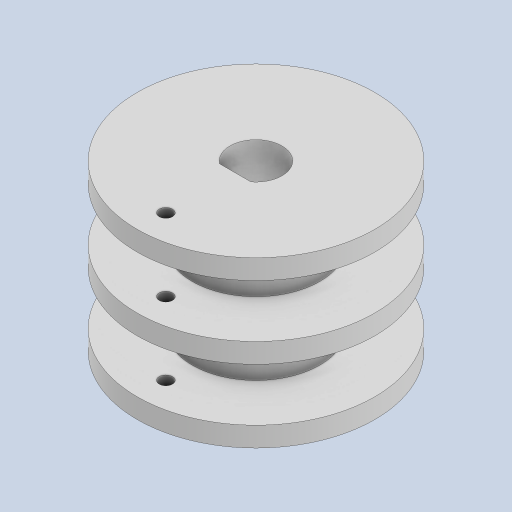
# Autodesk Inventor part: PulleyV2
Saved by Autodesk Inventor 2024 (Build 280153000, 153)
## iProperties
Created: 2024-01-01
Part Number: PulleyV2
Material: Generic
Document SubType Name: Modeling
Designer: Greg
Density: 1 g/cm^3
Appearance: Default
Author: Greg
Autodesk Inventor part; units mm, degrees
ref_plane "YZ Plane" through (0, 0, 0) normal (1, 0, 0) x (0, 1, 0)
ref_plane "XZ Plane" through (0, 0, 0) normal (0, 1, 0) x (-1, 0, 0)
ref_plane "XY Plane" through (0, 0, 0) normal (0, 0, 1) x (1, 0, 0)
sketch "Sketch1" plane through (0, 0, 0) normal (0, 1, 0) x (-1, 0, 0)
  circle A0 centre (0, 0) radius 14.2875
  dimension "d0" = 28.575
  constraints: 1 centre point, 1 coincident
  measures "d0" diameter of A0
extrude "Extrusion1" add sketch "Sketch1" along normal blind 2.3813
sketch "Sketch2" plane through (0, 2.3813, 0) normal (0, 1, 0) x (1, 0, 0)
  circle A0 centre (0, 0) radius 6.096 construction
  circle A1 centre (0, 0) radius 7.6835
  dimension "d6" = 12.192
  dimension "d7" = 1.5875
  constraints: 2 centre point, 1 coincident
  measures "d6" diameter of A0
  measures "d7" radial gap between concentric circles of A0 A1
extrude "Extrusion2" add sketch "Sketch2" along normal blind 6.35
sketch "Sketch3" plane through (0, 8.7313, 0) normal (0, 1, 0) x (1, 0, 0)
  circle A0 centre (0, 0) radius 14.2875
  circle A1 centre (0, 0) radius 14.2875 projected
  constraints: 1 centre point, 1 coincident, 1 concentric
extrude "Extrusion3" add sketch "Sketch3" along normal blind 2.3813
sketch "Sketch4" plane through (0, 11.1125, 0) normal (0, 1, 0) x (1, 0, 0)
  circle A0 centre (0, 0) radius 7.6835 projected
  circle A1 centre (0, 0) radius 7.6835
  constraints: 1 centre point, 1 coincident, 1 concentric
extrude "Extrusion4" add sketch "Sketch4" along normal blind 6.35
sketch "Sketch5" plane through (0, 17.4625, 0) normal (0, 1, 0) x (1, 0, 0)
  circle A0 centre (0, 0) radius 14.2875
  circle A1 centre (0, 0) radius 14.2875 projected
  constraints: 1 centre point, 1 coincident, 1 concentric
extrude "Extrusion5" add sketch "Sketch5" along normal blind 2.3813
sketch "Sketch6" plane through (0, 0, 0) normal (0, -1, 0) x (1, 0, 0)
  circle A0 centre (0, 0) radius 3.125
  line L0 (1.875, 2.5) -> (-1.875, 2.5)
  dimension "d16" = 6.25
  dimension "d35" = 2.5
  constraints: 2 end point, 2 point on circle, 1 centre point, 1 coincident, 1 horizontal
  measures "d16" diameter of A0
  measures "d35" distance from line of L0 point (0, 0)
extrude "Extrusion6" cut sketch "Sketch6" against normal through all contours A0 L0 picked at (0.5554, 0.5311)
sketch "Sketch7" plane through (0, 0, 0) normal (0, -1, 0) x (1, 0, 0)
  circle A0 centre (0, 0) radius 6.346
  dimension "d20" = 12.692
  constraints: 1 centre point, 1 coincident
  measures "d20" diameter of A0
extrude "Extrusion7" cut sketch "Sketch7" against normal blind 1.27
sketch "Sketch8" plane through (0, 0, 0) normal (0, -1, 0) x (1, 0, 0)
  circle A0 centre (0, 0) radius 3.125
  arc A1 (-1.875, 2.5) -> (1.875, 2.5) centre (0, 0) ccw projected
  constraints: 1 centre point, 1 coincident, 1 concentric
extrude "Extrusion8" cut sketch "Sketch8" against normal blind 4.445
sketch "Sketch9" plane through (0, 19.8438, 0) normal (0, 1, 0) x (1, 0, 0)
  circle A0 centre (0, 0) radius 7.6835 projected
  circle A1 centre (0, -10.8585) radius 0.7937
  point P0 (0, -7.6835)
  dimension "d31" = 1.5875
  dimension "d32" = 3.175
  constraints: 3 vertical alignment, 1 centre point, 1 other
  measures "d31" diameter of A1
  measures "d32" distance of point (0, -7.684) A1.centre
extrude "Extrusion9" cut sketch "Sketch9" against normal through all contours A1
equation "\"d10\" = d1"
equation "\"d12\" = d8"
equation "\"d14\" = d1"
equation "\"d18\" = d1"
equation "\"d1\" = 2.38125"
equation "\"d8\" = 6.35"
body "Solid1"
